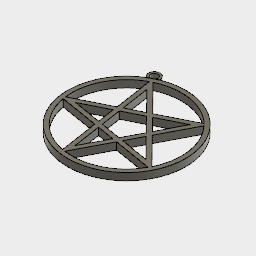
挂件 (Autodesk Fusion 360 design; units mm, degrees)
Autodesk Fusion 360 part; units mm, degrees
sketch "草图1" plane through (0, 0, 0) normal (0, 1, 0) x (1, 0, 0)
  circle A0 centre (0, 0) radius 40.6099
  line L0 (-13.7646, 7.1517) -> (-37.3253, -4.6183)
  line L1 (-13.2959, 4.0323) -> (-30.5587, -4.5915)
  line L2 (-17.6778, 33.1964) -> (-13.7646, 7.1517)
  line L3 (-13.8099, 27.6442) -> (-10.9427, 8.5614)
  line L4 (-13.2959, 4.0323) -> (-11.5238, -7.7615)
  line L5 (-11.0551, -10.8809) -> (-7.1419, -36.9256)
  line L6 (-10.474, 5.442) -> (-8.4123, -8.2797)
  line L7 (-7.9436, -11.3991) -> (-5.0764, -30.4819)
  line L8 (-30.5587, -4.5915) -> (-11.5238, -7.7615)
  line L9 (-37.0344, -6.5544) -> (-11.0551, -10.8809)
  line L10 (3.8206, -13.3583) -> (-5.0764, -30.4819)
  line L11 (6.9321, -13.8764) -> (-5.2107, -37.2472)
  line L12 (-8.4123, -8.2797) -> (5.2749, -10.5591)
  line L13 (8.3865, -11.0773) -> (27.4213, -14.2473)
  line L14 (-7.9436, -11.3991) -> (3.8206, -13.3583)
  line L15 (6.9321, -13.8764) -> (32.9114, -18.203)
  line L16 (13.8851, -0.4943) -> (27.4213, -14.2473)
  line L17 (15.3394, 2.3048) -> (33.814, -16.4657)
  line L18 (27.4822, 25.6755) -> (15.3394, 2.3048)
  line L19 (13.8851, -0.4943) -> (8.3865, -11.0773)
  line L20 (22.0237, 21.6765) -> (13.1267, 4.5529)
  line L21 (11.6724, 1.7538) -> (5.2749, -10.5591)
  line L22 (-15.9264, 34.0713) -> (2.5482, 15.3009)
  line L23 (4.7609, 13.0527) -> (13.1267, 4.5529)
  line L24 (-13.8099, 27.6442) -> (-0.2737, 13.8912)
  line L25 (1.939, 11.643) -> (11.6724, 1.7538)
  line L26 (26.1089, 27.0709) -> (2.5482, 15.3009)
  line L27 (-0.2737, 13.8912) -> (-10.9427, 8.5614)
  line L28 (22.0237, 21.6765) -> (4.7609, 13.0527)
  line L29 (1.939, 11.643) -> (-10.474, 5.442)
  arc A1 (33.814, -16.4657) -> (27.4822, 25.6755) centre (0, 0) ccw
  arc A2 (-5.2107, -37.2472) -> (32.9114, -18.203) centre (0, 0) ccw
  arc A3 (-37.0344, -6.5544) -> (-7.1419, -36.9256) centre (0, 0) ccw
  arc A4 (26.1089, 27.0709) -> (-15.9264, 34.0713) centre (0, 0) ccw
  arc A5 (-17.6778, 33.1964) -> (-37.3253, -4.6183) centre (0, 0) ccw
extrude "拉伸1" add sketch "草图1" along normal blind 5 makes body 1
sketch "草图2" plane through (0, 0, 0) normal (0, 1, 0) x (1, 0, 0)
  circle A0 centre (70, 0) radius 2.5
  circle A1 centre (70, 0) radius 4
  dimension "d6" = 5
  dimension "d7" = 8
  measures "d6" diameter of A0
  measures "d7" diameter of A1
extrude "拉伸2" add sketch "草图2" along normal blind 5 separate body makes body 2
move_body "移动1" bodies 2 to x (1, 0, 0) y (0, 1, 0) z (0, 0, 1) at (-89.4001, -0.2978, -38.4226)
combine "合并1" operation add target body 1 tool bodies 2
